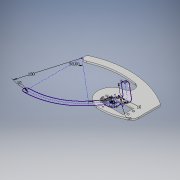
# Autodesk Inventor part: wstepna_geometria_wersja_2
Saved by Autodesk Inventor 2019 (Build 230136000, 136)
## iProperties
Created: 2022-02-09
Part Number: wstepna_geometria_wersja_2
Material: Generic
Document SubType Name: Modeling
Designer: Tomasz Krakowski
Density: 1 g/cm^3
Appearance: Default
Author: Tomasz Krakowski
Autodesk Inventor part; units mm, degrees
ref_plane "YZ Plane" through (0, 0, 0) normal (1, 0, 0) x (0, 1, 0)
ref_plane "XZ Plane" through (0, 0, 0) normal (0, 1, 0) x (-1, 0, 0)
ref_plane "XY Plane" through (0, 0, 0) normal (0, 0, 1) x (1, 0, 0)
sketch "Sketch1" plane through (0, 0, 0) normal (0, 1, 0) x (-1, 0, 0)
  arc A0 (-1.4142, 9.8995) -> (-10, 0) centre (0, 0) ccw
  line L0 (-39.5, 50) -> (0.5, 50)
  line L1 (0.5, 50) -> (0.5, 30)
  line L2 (0.5, 30) -> (-39.5, 30)
  line L3 (-39.5, 30) -> (-39.5, 50)
  line L4 (-39.5, 50) -> (0.5, 30) construction
  line L5 (0.5, 50) -> (-39.5, 30) construction
  line L6 (-10, 40) -> (-19.5, 40) construction
  circle A1 centre (4.5, 35.25) radius 1.9
  circle A2 centre (4.5, 44.75) radius 1.9
  line L7 (4.5, 44.75) -> (4.5, 35.25) construction
  circle A3 centre (-43.5, 44.75) radius 1.9
  circle A4 centre (-43.5, 35.25) radius 1.9
  line L8 (-43.5, 44.75) -> (-43.5, 35.25) construction
  line L9 (-43.5, 40) -> (-19.5, 40) construction
  line L10 (-10, 40) -> (4.5, 40) construction
  line L11 (-43.5, 44.75) -> (4.5, 44.75) construction
  line L12 (-43.5, 35.25) -> (4.5, 35.25) construction
  line L13 (-19.5, 40) -> (-19.5, 44.75) construction
  circle A5 centre (-10, 40) radius 9.75 construction
  circle A6 centre (-29, 40) radius 9.75 construction
  arc A7 (-2.7044, 60.2512) -> (-52.4397, 48.5007) centre (-10, -20) ccw
  arc A8 (-1.4142, 9.8995) -> (-2.7044, 60.2512) centre (-5, 35) ccw
  line L14 (-57.1731, 40) -> (-57.1731, 0)
  line L15 (-57.1731, 0) -> (0, 0) construction
  arc A9 (-52.4397, 48.5007) -> (-57.1731, 40) centre (-47.1731, 40) ccw
  line L16 (0, 0) -> (10, 0) construction
  line L17 (-10, 0) -> (-57.1731, 0) construction
  arc A10 (-10, 0) -> (-1.4142, -9.8995) centre (0, 0) ccw
  arc A11 (-1.8715, -9.8233) -> (77.546, -0.5248) centre (23.0596, 121.0399) ccw
  arc A12 (82.454, -11.4752) -> (77.546, -0.5248) centre (80, -6) ccw
  arc A13 (-57.1731, 0) -> (82.454, -11.4752) centre (23.0596, 121.0399) ccw
  line L18 (0, 0) -> (100, 0) construction
  point P0 (-57.1731, 45.3313)
  point P1 (-5, -35)
  dimension "d0" = 20
  dimension "d1" = 40
  dimension "d2" = 20
  dimension "d3" = 10.5
  dimension "d4" = 48
  dimension "d5" = 3.8
  dimension "d6" = 9.5
  dimension "d7" = 19.5
  dimension "d8" = 10
  dimension "d9" = 40
  dimension "d11" = 10.5
  dimension "d12" = 35
  dimension "d13" = 5
  dimension "d16" = 10
  dimension "d17" = 20
  dimension "d18" = 10
  dimension "d19" = 40
  dimension "d47" = 12
  dimension "d48" = 100
  dimension "d49" = 80
  constraints: 38 end point, 18 point on circle, 14 centre point, 8 tangent, 6 horizontal, 5 midpoint, 4 equal radius, 4 perpendicular, 3 coincident, 3 point on line, 2 collinear, 2 parallel, 2 symmetric about line, 2 vertical, 1 concentric, 1 other
  measures "d0" diameter of A0
  measures "d1" distance between parallel lines of L3 L1
  measures "d2" distance between parallel lines of L0 L2
  measures "d3" distance from line of L1 L6.start
  measures "d4" distance between parallel lines of L8 L7
  measures "d5" diameter of A1
  measures "d6" distance of L7.end L7.start
  measures "d7" diameter of A5
  measures "d8" horizontal distance of point (0, 0) L6.start
  measures "d9" vertical distance of point (0, 0) L6.start
  measures "d11" distance from line of L3 A6.centre
  measures "d12" vertical distance of point (0, 0) A8.centre
  measures "d13" horizontal distance of point (0, 0) A8.centre
  measures "d16" radius of A9
  measures "d17" vertical distance of point (0, 0) A7.centre
  measures "d18" horizontal distance of point (0, 0) A7.centre
  measures "d19" distance of L14.start L14.end
  measures "d47" diameter of A12
  measures "d48" distance of L18.end point (0, 0)
  measures "d49" horizontal distance of point (0, 0) A12.centre
extrude "Extrusion1" add sketch "Sketch1" along normal blind 3
sketch "Sketch2" plane through (0, 3, 0) normal (0, 1, 0) x (1, 0, 0)
  line L0 (10, -40) -> (-0.5, -40) construction
  line L1 (-0.5, -30) -> (-0.5, -50) construction
  line L2 (-0.5, -50) -> (-0.5, -30) construction
  line L3 (10, -40) -> (-9.2836, -62.9813) construction
  line L4 (15.1953, -18.2512) -> (-7.786, 1.0324) construction
  arc A0 (-85.8881, -98.7026) -> (-9.2836, -62.9813) centre (-85.8881, 1.2974) ccw construction
  line L5 (-9.2836, -62.9813) -> (-85.8881, 1.2974) construction
  line L6 (-85.8881, 1.2974) -> (-85.8881, -98.7026) construction
  line L7 (10, -40) -> (10, -30) construction
  line L8 (16.4279, -32.3396) -> (10, -40) construction
  arc A1 (16.4279, -32.3396) -> (15.1953, -18.2512) centre (8.7674, -25.9117) ccw construction
  line L9 (-0.5, -30) -> (39.5, -30) construction
  arc A2 (-85.8881, -93.7026) -> (-85.8881, -103.7026) centre (-85.8881, -98.7026) ccw
  arc A3 (-85.8881, -103.7026) -> (-5.4534, -66.1953) centre (-85.8881, 1.2974) ccw
  arc A4 (-85.8881, -93.7026) -> (-13.1139, -59.7674) centre (-85.8881, 1.2974) ccw
  line L10 (-9.2836, -62.9813) -> (-13.1139, -59.7674) construction
  line L11 (-9.2836, -62.9813) -> (-5.4534, -66.1953) construction
  line L12 (22.2395, -17.635) -> (-4.5721, 4.8626)
  arc A5 (-4.5721, 4.8626) -> (-11, -2.7978) centre (-7.786, 1.0324) ccw
  line L13 (8.1511, -18.8675) -> (-11, -2.7978)
  arc A6 (10.811, -22.3551) -> (8.1511, -18.8675) centre (1.7233, -26.528) ccw
  arc A7 (23.472, -31.7233) -> (22.2395, -17.635) centre (15.8116, -25.2954) ccw
  circle A8 centre (10, -40) radius 7 construction
  arc A9 (9.747, -50.9971) -> (20.7861, -37.8412) centre (10, -40) ccw
  arc A10 (7.4337, -29.3036) -> (-0.7861, -42.1588) centre (10, -40) ccw
  line L14 (-5.4534, -66.1953) -> (5.8018, -52.7818)
  line L15 (21.8586, -33.646) -> (23.472, -31.7233)
  line L16 (-13.1139, -59.7674) -> (-1.8586, -46.354)
  arc A11 (9.747, -50.9971) -> (5.8018, -52.7818) centre (9.632, -55.9958) ccw
  arc A12 (21.8586, -33.646) -> (20.7861, -37.8412) centre (25.6889, -36.86) ccw
  arc A13 (-1.8586, -46.354) -> (-0.7861, -42.1588) centre (-5.6889, -43.14) ccw
  arc A14 (7.4337, -29.3036) -> (10.811, -22.3551) centre (6.2671, -24.4415) ccw
  circle A15 centre (10, -40) radius 3
  point P0 (0, 0)
  point P1 (22.8558, -24.6791)
  point P2 (7.5322, -50.7196)
  point P3 (20.1282, -35.7083)
  dimension "d23" = 10.5
  dimension "d24" = 30
  dimension "d27" = 40
  dimension "d28" = 20
  dimension "d29" = 100
  dimension "d30" = 50
  dimension "d41" = 10
  dimension "d42" = 140
  dimension "d50" = 10
  dimension "d51" = 5
  dimension "d52" = 10
  dimension "d53" = 14
  dimension "d55" = 11
  dimension "d56" = 11
  dimension "d57" = 5
  dimension "d58" = 6
  constraints: 30 point on circle, 28 end point, 23 tangent, 16 centre point, 7 coincident, 6 perpendicular, 4 equal radius, 4 point on line, 2 collinear, 1 midpoint, 1 vertical, 2 other
  measures "d23" distance from line of L1 L0.start
  measures "d24" distance of L0.start L3.end
  measures "d27" distance of point (22.856, -24.679) L4.end
  measures "d28" distance of point (22.856, -24.679) L0.start
  measures "d29" radius of A0
  measures "d30" angle of L6 L5
  measures "d41" radius of A1
  measures "d42" angle of L7 L3
  measures "d50" diameter of A2
  measures "d51" radius of A5
  measures "d52" radius of A6
  measures "d53" diameter of A8
  measures "d55" radius of A10
  measures "d56" radius of A9
  measures "d57" radius of A11
  measures "d58" diameter of A15
equation "\"d11\" = d3"
body "Solid1"
